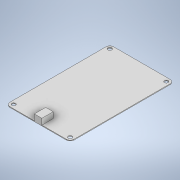
# Autodesk Inventor part: solar_panel
Saved by Autodesk Inventor 2022 (Build 260153000, 153)
## iProperties
Created: 2022-08-08
Part Number: solar_panel
Material: Generic
Document SubType Name: Modeling
Designer: thoma
Density: 1 g/cm^3
Appearance: Default
Author: thoma
Autodesk Inventor part; units mm, degrees
ref_plane "YZ Plane" through (0, 0, 0) normal (1, 0, 0) x (0, 1, 0)
ref_plane "XZ Plane" through (0, 0, 0) normal (0, 1, 0) x (-1, 0, 0)
ref_plane "XY Plane" through (0, 0, 0) normal (0, 0, 1) x (1, 0, 0)
sketch "Sketch1" plane through (0, 0, 0) normal (0, 1, 0) x (-1, 0, 0)
  line L0 (0, 0) -> (170, 0)
  line L1 (170, 0) -> (170, -275)
  line L2 (170, -275) -> (0, -275)
  line L3 (0, -275) -> (0, 0)
  dimension "d0" = 170
  dimension "d1" = 275
  constraints: 8 end point, 2 parallel, 1 horizontal, 1 perpendicular
  measures "d0" distance of L0.start L0.end
  measures "d1" distance of L2.end L0.start
extrude "Extrusion1" add sketch "Sketch1" along normal blind 2
fillet "Fillet1" radius 10 4 edges at (0, 1, 0) (-170, 1, 0) (0, 1, -275) (-170, 1, -275)
sketch "Sketch2" plane through (0, 2, 0) normal (0, 1, 0) x (1, 0, 0)
  line L0 (-160, 0) -> (-10, 0) projected
  line L1 (-75, 0) -> (-95, 0)
  line L2 (-95, 0) -> (-95, 30)
  line L3 (-95, 30) -> (-75, 30)
  line L4 (-75, 30) -> (-75, 0)
  line L5 (-85, 0) -> (-85, 30) construction
  line L6 (0, 10) -> (0, 265) construction
  point P0 (0, 0)
  dimension "d5" = 85
  dimension "d6" = 30
  dimension "d7" = 20
  constraints: 10 end point, 2 midpoint, 2 parallel, 1 horizontal, 1 perpendicular, 1 point on line
  measures "d5" distance between parallel lines of L6 L5
  measures "d6" distance of L3.end L1.start
  measures "d7" distance of L2.end L3.end
extrude "Extrusion2" add sketch "Sketch2" along normal blind 15.75
sketch "Sketch3" plane through (0, 0, 0) normal (0, -1, 0) x (1, 0, 0)
  line L0 (-160, 0) -> (-10, 0) construction
  line L1 (-85, 0) -> (-85, -25) construction
  line L2 (-160, -17.5) -> (-10, -17.5)
  line L3 (-10, -17.5) -> (-10, -32.5)
  line L4 (-10, -32.5) -> (-160, -32.5)
  line L5 (-160, -32.5) -> (-160, -17.5)
  line L6 (-160, -17.5) -> (-10, -32.5) construction
  line L7 (-10, -17.5) -> (-160, -32.5) construction
  line L8 (-51.7926, -17.5) -> (-51.7926, -32.5)
  line L9 (-47.6298, -32.5) -> (-47.6298, -17.5)
  line L10 (-102.3866, -17.5) -> (-102.3866, -32.5)
  line L11 (-107.5101, -32.5) -> (-107.5101, -17.5)
  point P0 (0, 0)
  dimension "d10" = 15
  dimension "d11" = 150
  dimension "d17" = 25
  constraints: 22 end point, 8 point on line, 5 perpendicular, 3 midpoint, 2 parallel, 1 horizontal, 1 vertical
  measures "d10" distance of L2.end L3.end
  measures "d11" distance of L2.start L2.end
  measures "d17" distance of L1.start L1.end
extrude "Extrusion3" cut sketch "Sketch3" against normal blind 0.3 contours L2 L11 L4 L5 | L2 L8 L4 L10 | L2 L3 L4 L9
pattern_linear "Rectangular Pattern1" count 12 spacing 20 along (0, 0, -1) of "Extrusion3"
sketch "Sketch4" plane through (0, 0, 0) normal (0, -1, 0) x (1, 0, 0)
  arc A0 (0, -10) -> (-10, 0) centre (-10, -10) ccw projected
  circle A1 centre (-10, -10) radius 5
  line L0 (0, -10) -> (0, -265) projected
  line L1 (-160, 0) -> (-10, 0) projected
  circle A2 centre (-10, -265) radius 5
  circle A3 centre (-160, -10) radius 5
  circle A4 centre (-160, -265) radius 5
  point P0 (0, 0)
  dimension "d18" = 10
  dimension "d21" = 255
  dimension "d24" = 150
  constraints: 4 centre point, 1 coincident, 1 horizontal, 1 vertical, 6 other
  measures "d18" diameter of A1
  measures "d21" distance of A1.centre A2.centre
  measures "d24" distance of A1.centre A3.centre
extrude "Extrusion4" cut sketch "Sketch4" against normal through all
equation "\"d5\" = 0.5 * d0"
body "Solid1"
